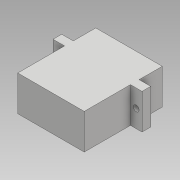
# Autodesk Inventor part: サーボ
Saved by Autodesk Inventor 2017 (Build 210142000, 142)
## iProperties
Part Number: サーボ
Material: 一般
Document SubType Name: Modeling
Designer: HISAAKI
Density: 1 g/cm^3
Appearance: 既定
Author: HISAAKI
Autodesk Inventor part; units mm, degrees
ref_plane "YZ Plane" through (0, 0, 0) normal (1, 0, 0) x (0, 1, 0)
ref_plane "XZ Plane" through (0, 0, 0) normal (0, 1, 0) x (-1, 0, 0)
ref_plane "XY Plane" through (0, 0, 0) normal (0, 0, 1) x (1, 0, 0)
sketch "スケッチ1" plane through (0, 0, 0) normal (0, 1, 0) x (-1, 0, 0)
  line L0 (0, 0) -> (23, 0)
  line L1 (23, 0) -> (23, -12.2)
  line L2 (23, -12.2) -> (0, -12.2)
  line L3 (0, -12.2) -> (0, 0)
  dimension "d0" = 23
  dimension "d1" = 12.2
  constraints: 8 end point, 2 parallel, 1 horizontal, 1 perpendicular
  measures "d0" distance of L1.end L2.end
  measures "d1" distance of L0.end L1.end
extrude "押し出し1" add sketch "スケッチ1" along normal blind 27
sketch "スケッチ2" plane through (0, 0, 0) normal (1, 0, 0) x (0, 0, -1)
  line L0 (0, 0) -> (0, 16)
  line L1 (0, 0) -> (0, 27) projected
  line L2 (0, 16) -> (12.2, 16)
  line L3 (12.2, 0) -> (12.2, 27) projected
  line L4 (0, 16) -> (0, 19)
  line L5 (0, 19) -> (12.2, 19)
  line L6 (12.2, 19) -> (12.2, 16)
  dimension "d4" = 16
  dimension "d5" = 3
  constraints: 10 end point, 3 perpendicular, 3 point on line
  measures "d4" distance of L0.start L0.end
  measures "d5" distance of L0.end L4.end
extrude "押し出し2" add sketch "スケッチ2" along normal blind 4
sketch "スケッチ3" plane through (-23, 0, -12.2) normal (-1, 0, 0) x (0, 0, 1)
  line L0 (0, 0) -> (0, 16.2076)
  line L1 (0, 16.2076) -> (12.2, 16.2076)
  line L2 (12.2, 16.2076) -> (12.2, 19.2076)
  line L3 (12.2, 19.2076) -> (0, 19.2076)
  line L4 (0, 0) -> (0, 27) projected
  line L5 (0, 19.2076) -> (0, 16.2076)
  point P0 (12.2, 0)
  dimension "d8" = 3
  constraints: 10 end point, 2 perpendicular, 1 collinear, 1 horizontal, 1 point on line, 1 vertical
  measures "d8" distance of L1.end L2.end
extrude "押し出し3" add sketch "スケッチ3" along normal blind 4
hole "穴2" at (-25, 19.2076, -6.1) direction (0, -1, 0) diameter 2 end through all
hole "穴3" at (2, 19, -6.1) direction (0, -1, 0) diameter 2 end through all
